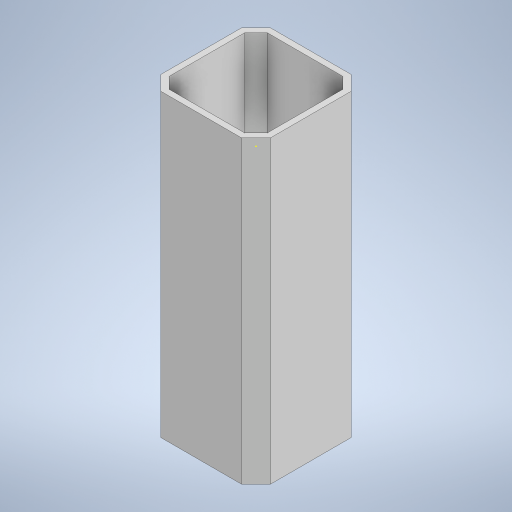
# Autodesk Inventor part: laser_leg
Saved by Autodesk Inventor 2024 (Build 280153000, 153)
## iProperties
Created: 2024-04-21
Part Number: laser_leg
Material: Generic
Document SubType Name: Modeling
Designer: kamil
Density: 1 g/cm^3
Appearance: Default
Author: kamil
Autodesk Inventor part; units mm, degrees
ref_plane "YZ Plane" through (0, 0, 0) normal (1, 0, 0) x (0, 1, 0)
ref_plane "XZ Plane" through (0, 0, 0) normal (0, 1, 0) x (-1, 0, 0)
ref_plane "XY Plane" through (0, 0, 0) normal (0, 0, 1) x (1, 0, 0)
sketch "Sketch1" plane through (0, 0, 0) normal (0, 1, 0) x (-1, 0, 0)
  line L0 (65, 0) -> (10, 0)
  line L1 (0, -10) -> (0, -65)
  line L2 (10, -75) -> (65, -75)
  line L3 (75, -65) -> (75, -10)
  line L4 (75, -10) -> (65, 0)
  line L5 (10, 0) -> (0, -10)
  line L6 (0, -65) -> (10, -75)
  line L7 (75, -65) -> (65, -75)
  point P0 (0, 0)
  point P1 (75, 0)
  point P2 (0, -75)
  point P3 (0, 0)
  point P4 (75, -75)
  dimension "d0" = 75
  dimension "d1" = 75
  dimension "d2" = 10
  dimension "d3" = 10
  dimension "d4" = 10
  dimension "d5" = 10
  dimension "d6" = 10
  dimension "d7" = 10
  dimension "d8" = 10
  dimension "d9" = 10
  constraints: 16 end point, 8 point on line, 2 parallel, 1 coincident, 1 horizontal, 1 perpendicular
  measures "d0" distance of point (0, 0) point (0, -75)
  measures "d1" distance of point (0, -75) point (75, -75)
  measures "d2" distance of L3.end point (75, 0)
  measures "d3" distance of L0.start point (75, 0)
  measures "d4" distance of L0.end point (0, 0)
  measures "d5" distance of L1.start point (0, 0)
  measures "d6" distance of L1.end point (0, -75)
  measures "d7" distance of L2.start point (0, -75)
  measures "d8" distance of L3.start point (75, -75)
  measures "d9" distance of L2.end point (75, -75)
extrude "Extrusion1" add sketch "Sketch1" along normal blind 5
sketch "Sketch2" plane through (0, 5, 0) normal (0, 1, 0) x (1, 0, 0)
  line L0 (-75, 10) -> (-65, 0) projected
  line L1 (-75, 65) -> (-75, 10) projected
  line L2 (-75, 10) -> (-75, 65)
  line L3 (-65, 75) -> (-75, 65) projected
  line L4 (-75, 65) -> (-65, 75)
  line L5 (-75, 10) -> (-65, 0)
  line L6 (-65, 0) -> (-10, 0) projected
  line L7 (-10, 0) -> (0, 10) projected
  line L8 (-10, 0) -> (0, 10)
  line L9 (0, 10) -> (0, 65) projected
  line L10 (0, 10) -> (0, 65)
  line L11 (0, 65) -> (-10, 75)
  line L12 (-10, 75) -> (-65, 75) projected
  line L13 (-10, 75) -> (-65, 75)
  line L14 (-65, 0) -> (-10, 0)
  line L15 (-11.6569, 71) -> (-4, 63.3431)
  line L16 (-4, 63.3431) -> (-4, 11.6569)
  line L17 (-4, 11.6569) -> (-11.6569, 4)
  line L18 (-11.6569, 4) -> (-63.3431, 4)
  line L19 (-63.3431, 4) -> (-71, 11.6569)
  line L20 (-71, 11.6569) -> (-71, 63.3431)
  line L21 (-71, 63.3431) -> (-63.3431, 71)
  line L22 (-63.3431, 71) -> (-11.6569, 71)
  point P0 (0, 0)
  dimension "d12" = 4
  constraints: 32 end point, 6 collinear, 2 perpendicular, 1 point on line, 7 other
  measures "d12" distance between parallel lines of L11 L15
extrude "Extrusion2" add sketch "Sketch2" along normal blind 200
sketch "Sketch3" plane through (-10, 0, -75) normal (0, 0, -1) x (-1, 0, 0)
  circle A0 centre (27.5, 20) radius 5
  line L0 (0, 0) -> (0, 205) construction
  line L1 (55, 0) -> (0, 0) construction
  line L2 (0, 0) -> (55, 0) construction
  point P0 (-10, 0)
  point P1 (27.5, 0)
  dimension "d15" = 10
  dimension "d16" = 20
  dimension "d17" = 55
  dimension "d18" = 27.5
  constraints: 2 end point, 1 centre point, 1 collinear, 1 midpoint
  measures "d15" diameter of A0
  measures "d16" distance of point (27.5, 0) A0.centre
  measures "d17" distance of L1.start L0.start
  measures "d18" distance from line of L0 A0.centre
extrude "Extrusion3" cut sketch "Sketch3" against normal blind 4
sketch "Sketch4" plane through (0, 205, 0) normal (0, 1, 0) x (1, 0, 0)
  point P0 (0, 0)
equation "\"d3\" = d2"
equation "\"d4\" = d2"
equation "\"d5\" = d4"
equation "\"d6\" = d2"
equation "\"d7\" = d6"
equation "\"d8\" = d2"
equation "\"d9\" = d8"
body "Solid1"
